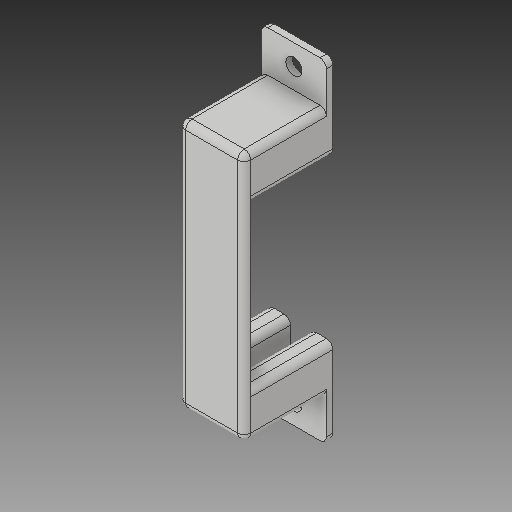
# Autodesk Inventor part: BackWheelServoClasp
Saved by Autodesk Inventor 2018 (Build 220112000, 112)
## iProperties
Created: 2017-11-24
Part Number: BackWheelServoClasp
Material: Generic
Document SubType Name: Modeling
Designer: reide
Density: 1 g/cm^3
Appearance: Default
Author: reide
Autodesk Inventor part; units mm, degrees
ref_plane "YZ Plane" through (0, 0, 0) normal (1, 0, 0) x (0, 1, 0)
ref_plane "XZ Plane" through (0, 0, 0) normal (0, 1, 0) x (-1, 0, 0)
ref_plane "XY Plane" through (0, 0, 0) normal (0, 0, 1) x (1, 0, 0)
sketch "Sketch1" plane through (0, 0, 0) normal (0, 0, 1) x (1, 0, 0)
  line L0 (93.893, 28.1705) -> (89.575, 28.1705) projected
  line L1 (89.575, 12.9305) -> (89.575, 28.1705) projected
  line L2 (89.575, 7.8505) -> (89.575, 12.9305) projected
  line L3 (93.893, 7.8505) -> (89.575, 7.8505) projected
  line L4 (93.893, 7.8505) -> (93.893, 2.0085) projected
  line L5 (93.893, 2.0085) -> (96.433, 2.0085) projected
  line L6 (96.433, 7.8505) -> (96.433, 2.0085) projected
  line L7 (112.435, 7.8505) -> (96.433, 7.8505) projected
  line L8 (112.435, 7.8505) -> (112.435, 28.1705) projected
  line L9 (112.435, 28.1705) -> (96.433, 28.1705) projected
  line L10 (96.433, 34.0125) -> (96.433, 28.1705) projected
  line L11 (93.893, 34.0125) -> (96.433, 34.0125) projected
  line L12 (93.893, 34.0125) -> (93.893, 28.1705) projected
  line L13 (93.893, 6.5805) -> (89.575, 6.5805) projected
  line L14 (112.435, 6.5805) -> (96.433, 6.5805) projected
  line L15 (93.893, 29.4405) -> (89.575, 29.4405) projected
  line L16 (112.435, 29.4405) -> (96.433, 29.4405) projected
  line L17 (93.893, 6.5805) -> (93.643, 6.5805)
  line L18 (93.643, 6.5805) -> (93.643, 2.0085)
  line L19 (93.643, 2.0085) -> (93.643, 1.7585)
  line L20 (93.643, 1.7585) -> (90.143, 1.7585)
  line L21 (90.143, 1.7585) -> (90.143, 6.5805)
  line L22 (95.163, 2.0085) -> (95.163, 1.3114)
  line L23 (96.683, 6.5805) -> (96.683, 2.0085)
  line L24 (96.683, 2.0085) -> (96.683, 1.7585)
  line L25 (96.683, 1.7585) -> (100.183, 1.7585)
  line L26 (100.183, 1.7585) -> (100.183, 6.5805)
  line L27 (90.143, 1.7585) -> (100.183, 1.7585)
  line L28 (100.183, 1.7585) -> (100.183, -1.2415)
  line L29 (100.183, -1.2415) -> (90.143, -1.2415)
  line L30 (90.143, -1.2415) -> (90.143, 1.7585)
  line L31 (112.435, 18.0105) -> (108.4742, 18.0105)
  line L32 (93.893, 28.1705) -> (93.893, 34.0125)
  line L33 (93.893, 34.0125) -> (96.433, 34.0125)
  line L34 (96.433, 28.1705) -> (96.433, 34.0125)
  line L35 (112.435, 6.5805) -> (96.433, 6.5805)
  line L36 (93.643, 29.4405) -> (93.643, 34.0125)
  line L37 (93.643, 34.0125) -> (93.643, 34.2625)
  line L38 (93.643, 34.2625) -> (90.143, 34.2625)
  line L39 (90.143, 34.2625) -> (90.143, 29.4405)
  line L40 (95.163, 34.0125) -> (95.163, 34.7096)
  line L41 (96.683, 29.4405) -> (96.683, 34.0125)
  line L42 (100.183, 34.2625) -> (100.183, 29.4405)
  line L43 (96.683, 34.0125) -> (96.683, 34.2625)
  line L44 (96.683, 34.2625) -> (100.183, 34.2625)
  line L45 (90.143, 34.2625) -> (100.183, 34.2625)
  line L46 (100.183, 34.2625) -> (100.183, 37.2625)
  line L47 (100.183, 37.2625) -> (90.143, 37.2625)
  line L48 (90.143, 37.2625) -> (90.143, 34.2625)
  line L49 (96.683, 6.5805) -> (100.183, 6.5805)
  line L50 (100.183, 6.5805) -> (100.183, -1.2415)
  line L51 (100.183, -1.2415) -> (96.683, -1.2415)
  line L52 (96.683, -1.2415) -> (96.683, 6.5805)
  line L53 (96.683, 29.4405) -> (100.183, 29.4405)
  line L54 (100.183, 29.4405) -> (100.183, 37.2625)
  line L55 (100.183, 37.2625) -> (96.683, 37.2625)
  line L56 (96.683, 37.2625) -> (96.683, 29.4405)
  line L57 (90.143, 29.4405) -> (93.643, 29.4405)
  line L58 (93.643, 29.4405) -> (93.643, 37.2625)
  line L59 (93.643, 37.2625) -> (90.143, 37.2625)
  line L60 (90.143, 37.2625) -> (90.143, 29.4405)
  point P0 (0, 0)
  dimension "d0" = 0.25
  dimension "d1" = 0.25
  dimension "d2" = 3.5
  dimension "d3" = 3
  constraints: 88 end point, 20 symmetric about line, 8 parallel, 7 point on line, 6 perpendicular, 5 horizontal, 2 midpoint, 2 vertical
  measures "d0" distance of L13.start L17.end
  measures "d1" distance of L18.end L19.end
  measures "d2" distance of L19.end L20.end
  measures "d3" distance of L27.end L28.end
extrude "Extrusion1" add sketch "Sketch1" along normal blind 12.7 contours L15 L39 L38 L37 L36 | L45 L58 L47 L56 | L48 L47 L58 L38 | L44 L42 L16 L41 L43 | L56 L47 L46 L44 | L18 L19 L20 L21 L13 | L27 L52 L29 L30 L20 | L24 L23 L14 L26 L25 | L25 L28 L29 L52
sketch "Sketch2" plane through (0, 0, 12.7) normal (0, 0, 1) x (1, 0, 0)
  line L0 (90.143, 6.5805) -> (90.143, -1.2415) projected
  line L1 (100.183, 29.4405) -> (100.183, 37.2625) projected
  line L2 (90.143, -1.2415) -> (100.183, -1.2415)
  line L3 (100.183, -1.2415) -> (100.183, 37.2625)
  line L4 (100.183, 37.2625) -> (90.143, 37.2625)
  line L5 (90.143, 37.2625) -> (90.143, -1.2415)
  point P0 (0, 0)
  constraints: 8 end point, 2 parallel, 1 horizontal, 1 perpendicular
extrude "Extrusion2" add sketch "Sketch2" along normal blind 1
sketch "Sketch3" plane through (0, 0, 0) normal (0, 0, -1) x (-1, 0, 0)
  line L0 (-90.143, -1.2415) -> (-100.183, -1.2415) projected
  line L1 (-100.183, 37.2625) -> (-90.143, 37.2625) projected
  line L2 (-90.143, -1.2415) -> (-100.183, -1.2415)
  line L3 (-100.183, -1.2415) -> (-100.183, -7.5915)
  line L4 (-100.183, -7.5915) -> (-90.143, -7.5915)
  line L5 (-90.143, -7.5915) -> (-90.143, -1.2415)
  line L6 (-100.183, 29.4405) -> (-100.183, 37.2625) projected
  line L7 (-100.183, 37.2625) -> (-90.143, 37.2625)
  line L8 (-90.143, 37.2625) -> (-90.143, 43.6125)
  line L9 (-90.143, 43.6125) -> (-100.183, 43.6125)
  line L10 (-100.183, 43.6125) -> (-100.183, 37.2625)
  circle A0 centre (-95.163, -4.4165) radius 1.25
  circle A1 centre (-95.163, 40.4375) radius 1.25
  point P0 (0, 0)
  point P1 (-90.143, -4.4165)
  point P2 (-90.143, 40.4375)
  point P3 (-95.163, 43.6125)
  point P4 (-95.163, -7.5915)
  dimension "d8" = 6.35
  dimension "d9" = 6.35
  dimension "d10" = 2.5
  dimension "d11" = 2.5
  constraints: 16 end point, 4 midpoint, 4 parallel, 2 centre point, 2 horizontal, 2 perpendicular, 1 point on line
  measures "d8" distance of L7.end L8.end
  measures "d9" distance of L4.end L0.start
  measures "d10" diameter of A0
  measures "d11" diameter of A1
extrude "Extrusion3" add sketch "Sketch3" against normal blind 1
fillet "Fillet2" radius 1 4 edges at (90.143, 43.6125, 0.5) (100.183, 43.6125, 0.5) (90.143, -7.5915, 0.5) (100.183, -7.5915, 0.5)
sketch "Sketch4" plane through (0, 0, 0) normal (0, 0, -1) x (-1, 0, 0)
  line L0 (-100.183, 6.5805) -> (-96.683, 6.5805) projected
  line L1 (-96.683, 6.5805) -> (-96.683, 5.5805)
  line L2 (-96.683, 6.5805) -> (-96.683, 1.7585) projected
  line L3 (-96.683, 5.5805) -> (-100.1874, 5.5805)
  line L4 (-100.1874, 5.5805) -> (-100.1874, 6.5805)
  line L5 (-100.1874, 6.5805) -> (-96.683, 6.5805)
  line L6 (-94.143, 2.0085) -> (-94.143, 7.8505) projected
  line L7 (-94.143, 6.5805) -> (-89.825, 6.5805) projected
  line L8 (-90.143, 29.4405) -> (-90.143, 6.5805) projected
  line L9 (-94.143, 5.5805) -> (-90.143, 5.5805)
  line L10 (-90.143, 5.5805) -> (-90.143, 6.5805)
  line L11 (-90.143, 6.5805) -> (-94.143, 6.5805)
  line L12 (-94.143, 6.5805) -> (-94.143, 5.5805)
  line L13 (-100.183, 6.5805) -> (-100.183, 29.4405) projected
  line L14 (-100.183, 18.0105) -> (-103.7607, 18.0105)
  line L15 (-100.183, 29.4405) -> (-96.683, 29.4405)
  line L16 (-96.683, 29.4405) -> (-96.683, 30.4405)
  line L17 (-96.683, 29.4405) -> (-96.683, 34.2625)
  line L18 (-96.683, 30.4405) -> (-100.1874, 30.4405)
  line L19 (-100.1874, 30.4405) -> (-100.1874, 29.4405)
  line L20 (-100.1874, 29.4405) -> (-96.683, 29.4405)
  line L21 (-94.143, 34.0125) -> (-94.143, 28.1705)
  line L22 (-94.143, 29.4405) -> (-89.825, 29.4405)
  line L23 (-90.143, 6.5805) -> (-90.143, 29.4405)
  line L24 (-94.143, 30.4405) -> (-90.143, 30.4405)
  line L25 (-90.143, 30.4405) -> (-90.143, 29.4405)
  line L26 (-90.143, 29.4405) -> (-94.143, 29.4405)
  line L27 (-94.143, 29.4405) -> (-94.143, 30.4405)
  line L28 (-100.183, 29.4405) -> (-100.183, 6.5805)
  point P0 (0, 0)
  dimension "d17" = 1
  dimension "d23" = 1
  constraints: 46 end point, 16 symmetric about line, 4 perpendicular, 4 point on line, 2 horizontal, 2 parallel, 1 midpoint
  measures "d17" distance of L0.end L1.end
  measures "d23" distance between parallel lines of L9 L7
extrude "Extrusion4" cut sketch "Sketch4" against normal up to surface (12.7 mm away)
fillet "Fillet4" radius 1 8 edges at (96.683, 5.5805, 6.35) (100.183, 5.5805, 6.35) (93.643, 5.5805, 6.35) (90.143, 5.5805, 6.35) (100.183, 30.4405, 6.35) (96.683, 30.4405, 6.35) (93.643, 30.4405, 6.35) (90.143, 30.4405, 6.35)
fillet "Fillet5" radius 1 4 edges at (100.183, -1.2415, 7.35) (90.143, -1.2415, 7.35) (100.183, 37.2625, 7.35) (90.143, 37.2625, 7.35)
fillet "Fillet6" radius 1 8 edges at (90.4359, -0.9486, 13.7) (95.163, -1.2415, 13.7) (99.8901, -0.9486, 13.7) (100.183, 18.0105, 13.7) (99.8901, 36.9696, 13.7) (95.163, 37.2625, 13.7) (90.4359, 36.9696, 13.7) (90.143, 18.0105, 13.7)
sketch "Sketch5" plane through (0, 0, 0) normal (0, 0, -1) x (-1, 0, 0)
  line L0 (-96.683, 1.7585) -> (-93.643, 1.7585) projected
  line L1 (-96.683, 1.7585) -> (-93.643, 1.7585)
  line L2 (-93.643, 1.7585) -> (-93.643, 1.2585)
  line L3 (-93.643, 1.2585) -> (-96.683, 1.2585)
  line L4 (-96.683, 1.2585) -> (-96.683, 1.7585)
  line L5 (-100.183, 4.5805) -> (-100.183, 31.4405) projected
  line L6 (-100.183, 18.0105) -> (-106.4704, 18.0105)
  line L7 (-96.683, 34.2625) -> (-93.643, 34.2625)
  line L8 (-96.683, 34.2625) -> (-93.643, 34.2625)
  line L9 (-93.643, 34.2625) -> (-93.643, 34.7625)
  line L10 (-93.643, 34.7625) -> (-96.683, 34.7625)
  line L11 (-96.683, 34.7625) -> (-96.683, 34.2625)
  point P0 (0, 0)
  dimension "d24" = 0.5
  constraints: 20 end point, 5 symmetric about line, 2 horizontal, 2 parallel, 1 midpoint, 1 perpendicular
  measures "d24" distance of L3.end L0.start
extrude "Extrusion5" cut sketch "Sketch5" against normal up to surface (12.7 mm away)
body "Solid1"
